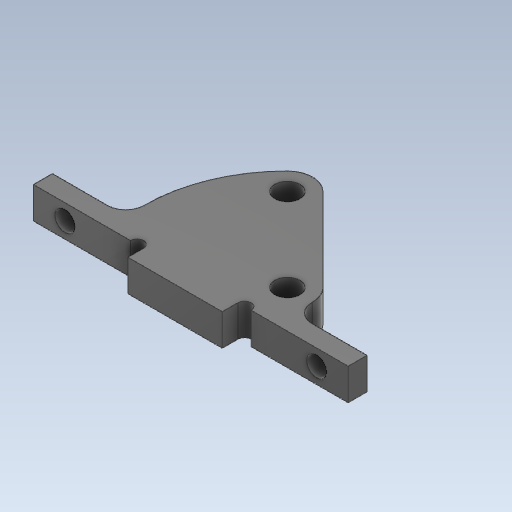
# Autodesk Inventor part: Camera_side_frame
Saved by Autodesk Inventor 2020.4 (Build 244396000, 396)
## iProperties
Part Number: Camera_side_frame
Material: アセタール樹脂、黒
Document SubType Name: Modeling
Designer: Masato Kubotera
Density: 1.425 g/cm^3
Appearance: 滑らか - 黒
Mass: 4.21188 g
Surface Area: 20.6112 cm^2
Volume: 2.95571 cm^3
Description: POM T5
Author: Masato Kubotera
Autodesk Inventor part; units mm, degrees
ref_plane "YZ Plane" through (0, 0, 0) normal (1, 0, 0) x (0, 1, 0)
ref_plane "XZ Plane" through (0, 0, 0) normal (0, 1, 0) x (-1, 0, 0)
ref_plane "XY Plane" through (0, 0, 0) normal (0, 0, 1) x (1, 0, 0)
derived "Head_basis.ipt"
sketch "スケッチ1" plane through (0, 0, 0) normal (0, 1, 0) x (-1, 0, 0)
  line L0 (-44.985, 68.48) -> (-70.7944, 42.6706) construction
  line L1 (4.795, 25.7) -> (-9.205, 25.7) construction
  line L2 (-2.205, 25.7) -> (-44.985, 68.48) construction
  line L3 (-2.205, 25.7) -> (-2.205, 4.9887) construction
  line L4 (-54.1774, 48.681) -> (-57.7129, 52.2165) construction
  line L5 (-57.7129, 52.2165) -> (-80.3403, 29.5891) construction
  line L6 (-80.3403, 29.5891) -> (-76.8048, 26.0536) construction
  line L7 (-76.8048, 26.0536) -> (-54.1774, 48.681) construction
  line L8 (-54.1774, 48.681) -> (-80.3403, 29.5891) construction
  line L9 (-57.7129, 52.2165) -> (-76.8048, 26.0536) construction
  line L10 (-61.9555, 44.4383) -> (-72.5621, 33.8317) construction
  line L11 (-70.7944, 32.064) -> (-60.1878, 42.6706) construction
  circle A0 centre (-59.4807, 46.9132) radius 1.6 construction
  line L12 (-55.9451, 50.4487) -> (-78.5725, 27.8213) construction
  line L13 (17.795, -2.5) -> (-22.205, -2.5) construction
  line L14 (3.8601, -2.5) -> (3.8601, 2.5) construction
  line L15 (5.295, -2.5) -> (5.295, 0)
  line L16 (10.8483, 2.5) -> (7.6861, 2.5) construction
  line L17 (-9.705, -2.5) -> (-9.705, 0)
  line L18 (5.6869, 2.5) -> (7.6861, 2.5) construction
  line L19 (-18.705, 0.5) -> (-16.205, 0.5) construction
  line L20 (-24.705, -2.5) -> (20.295, -2.5) construction
  arc A1 (5.295, -2.5) -> (7.395, -2.5) centre (6.345, -2.5) ccw
  line L21 (9.935, -2.5) -> (11.935, -2.5) construction
  line L22 (7.395, -2.5) -> (22.795, -2.5)
  line L23 (22.795, -2.5) -> (22.795, -5.5)
  line L24 (22.795, -5.5) -> (14.045, -5.5)
  line L25 (17.795, -2.5) -> (17.795, -5.5) construction
  arc A2 (-11.805, -2.5) -> (-9.705, -2.5) centre (-10.755, -2.5) ccw
  line L26 (-11.805, -2.5) -> (-27.205, -2.5)
  line L27 (-27.205, -2.5) -> (-27.205, -5.5)
  line L28 (-22.205, -2.5) -> (-22.205, -5.5) construction
  line L29 (-18.455, -5.5) -> (-27.205, -5.5)
  circle A3 centre (-11.5482, -8.5) radius 2
  arc A4 (14.045, -5.5) -> (11.1379, -8.4177) centre (14.045, -8.4071) ccw
  line L30 (15.045, -5.5) -> (15.045, -6.9) construction
  line L31 (15.045, -6.9) -> (20.545, -6.9) construction
  line L32 (20.545, -5.5) -> (20.545, -6.9) construction
  circle A5 centre (-11.5482, -8.5) radius 4
  line L33 (22.795, -2.5) -> (22.795, 0.5)
  line L34 (-2.205, -12.0113) -> (-2.205, 4.9887) construction
  line L35 (-19.455, -5.5) -> (-19.455, -6.9) construction
  line L36 (-19.455, -6.9) -> (-24.955, -6.9) construction
  line L37 (-24.955, -5.5) -> (-24.955, -6.9) construction
  line L38 (-69.0266, 40.9028) -> (-65.4911, 37.3673) construction
  circle A6 centre (-75.037, 31.3569) radius 1.6
  line L39 (-32.205, -2.5) -> (-22.205, -2.5)
  circle A7 centre (1.665, -21.7132) radius 2
  arc A8 (4.4934, -24.5416) -> (11.1379, -8.4177) centre (-11.5482, -8.5) ccw
  line L40 (-14.3767, -11.3284) -> (-1.1635, -24.5416)
  circle A9 centre (1.665, -21.7132) radius 4
  line L41 (4.4934, -18.8848) -> (-8.7198, -5.6716)
  line L42 (1.665, -21.7132) -> (-11.5482, -8.5) construction
  line L43 (-49.2969, -22.1777) -> (-31.6192, -4.5) construction
  line L44 (-31.6192, -4.5) -> (-28.0837, -8.0355) construction
  line L45 (-28.0837, -8.0355) -> (-45.7614, -25.7132) construction
  line L46 (-45.7614, -25.7132) -> (-49.2969, -22.1777) construction
  line L47 (-49.2969, -22.1777) -> (-28.0837, -8.0355) construction
  line L48 (-31.6192, -4.5) -> (-45.7614, -25.7132) construction
  line L49 (-47.5291, -23.9454) -> (-29.8515, -6.2678) construction
  line L50 (-40.4581, -13.3388) -> (-36.9225, -16.8744) construction
  line L51 (-40.1045, -20.0563) -> (-33.7405, -13.6924) construction
  line L52 (-33.7405, -13.6924) -> (-37.2761, -10.1569) construction
  line L53 (-37.2761, -10.1569) -> (-43.64, -16.5208) construction
  line L54 (-43.64, -16.5208) -> (-40.1045, -20.0563) construction
  line L55 (-40.1045, -20.0563) -> (-37.2761, -10.1569) construction
  line L56 (-33.7405, -13.6924) -> (-43.64, -16.5208) construction
  circle A10 centre (-45.4078, -21.8241) radius 1.6
  line L57 (-42.2258, -15.0359) -> (-38.761, -11.5711)
  line L58 (-37.2761, -10.0861) -> (-33.6698, -13.6924)
  line L59 (-35.1548, -15.1773) -> (-38.6196, -18.6421)
  line L60 (-40.1045, -20.1271) -> (-43.7107, -16.5208)
  line L61 (-43.7107, -16.5208) -> (-33.6698, -13.6924) construction
  line L62 (-37.2761, -10.0861) -> (-40.1045, -20.1271) construction
  arc A11 (-42.2258, -15.0359) -> (-43.7107, -16.5208) centre (-42.9683, -15.7784) ccw
  arc A12 (-37.2761, -10.0861) -> (-38.761, -11.5711) centre (-38.0185, -10.8286) ccw
  circle A13 centre (-31.9728, -8.3891) radius 1.6
  line L63 (-41.8723, -18.2886) -> (-35.5083, -11.9246) construction
  arc A14 (-40.1045, -20.1271) -> (-38.6196, -18.6421) centre (-39.362, -19.3846) ccw
  arc A15 (-35.1548, -15.1773) -> (-33.6698, -13.6924) centre (-34.4123, -14.4349) ccw
  line L64 (-32.205, 19.5) -> (-24.205, 27.5)
  circle A16 centre (-32.205, -2.5) radius 1 construction
  line L65 (-11.5482, -4.5) -> (-31.6192, -4.5)
  line L66 (-57.7129, 52.2165) -> (-54.1774, 48.681)
  line L67 (-76.8048, 26.0536) -> (-80.3403, 29.5891)
  line L68 (-80.3403, 29.5891) -> (-57.7129, 52.2165)
  line L69 (-45.7614, -25.7132) -> (1.665, -25.7132)
  line L70 (-45.7614, -25.7132) -> (-49.2969, -22.1777)
  arc A17 (-15.5479, -8.4464) -> (-18.455, -5.5) centre (-18.455, -8.4074) ccw
  line L71 (-49.2969, 13.1777) -> (-45.7614, 9.6421) construction
  line L72 (-45.7614, 9.6421) -> (-63.439, -8.0355) construction
  line L73 (-49.2969, 13.1777) -> (-63.439, -8.0355) construction
  arc A18 (-59.9035, 2.6418) -> (-61.3884, 1.1569) centre (-60.646, 1.8993) ccw
  line L74 (-52.8324, 2.5004) -> (-56.2972, -0.9645)
  line L75 (-57.7822, -2.4494) -> (-61.3884, 1.1569)
  line L76 (-61.3177, 1.1569) -> (-57.7822, -2.3787) construction
  line L77 (-66.9746, -4.5) -> (-49.2969, 13.1777) construction
  line L78 (-58.1357, 4.3388) -> (-54.6002, 0.8033) construction
  arc A19 (-57.7822, -2.4494) -> (-56.2972, -0.9645) centre (-57.0397, -1.7069) ccw
  line L79 (-59.5499, -0.6109) -> (-53.186, 5.753) construction
  line L80 (-59.9035, 2.6418) -> (-56.4387, 6.1066)
  line L81 (-51.4182, 3.9853) -> (-61.3177, 1.1569) construction
  line L82 (-61.3884, 1.1569) -> (-51.3475, 3.9853) construction
  arc A20 (-52.8324, 2.5004) -> (-51.3475, 3.9853) centre (-52.09, 3.2428) ccw
  line L83 (-57.7822, -2.3787) -> (-51.4182, 3.9853) construction
  line L84 (-54.9537, 7.5208) -> (-61.3177, 1.1569) construction
  arc A21 (-54.9537, 7.5915) -> (-56.4387, 6.1066) centre (-55.6962, 6.8491) ccw
  line L85 (-57.7822, -2.3787) -> (-54.9537, 7.5208) construction
  line L86 (-51.4182, 3.9853) -> (-54.9537, 7.5208) construction
  line L87 (-54.9537, 7.5915) -> (-51.3475, 3.9853)
  circle A22 centre (-49.6504, 9.2886) radius 1.6
  line L88 (-66.9746, -4.5) -> (-45.7614, 9.6421) construction
  line L89 (-65.2068, -6.2678) -> (-47.5291, 11.4099) construction
  line L90 (-54.9537, 7.5915) -> (-57.7822, -2.4494) construction
  line L91 (-63.439, -8.0355) -> (-66.9746, -4.5) construction
  circle A23 centre (-63.0855, -4.1464) radius 1.6
  line L92 (-63.439, -8.0355) -> (-66.9746, -4.5)
  line L93 (-31.6192, -4.5) -> (-45.7614, 9.6421)
  line L94 (-49.2969, 13.1777) -> (-45.7614, 9.6421)
  line L95 (-49.2969, 13.1777) -> (-54.1774, 48.681)
  line L96 (-76.8048, 26.0536) -> (-66.9746, -4.5)
  line L97 (-63.439, -8.0355) -> (-49.2969, -22.1777)
  line L98 (-54.1774, 48.681) -> (-76.8048, 26.0536) construction
  line L99 (-57.2115, 34.0383) -> (-54.7238, 15.9412)
  line L100 (-55.291, 14.2547) -> (-62.4067, 7.139)
  line L101 (-65.7248, 7.9406) -> (-70.7355, 23.5147)
  line L102 (-70.2458, 25.5414) -> (-60.6071, 35.1802)
  arc A24 (-57.2115, 34.0383) -> (-60.6071, 35.1802) centre (-59.1929, 33.7659) ccw
  arc A25 (-70.2458, 25.5414) -> (-70.7355, 23.5147) centre (-68.8316, 24.1272) ccw
  arc A26 (-65.7248, 7.9406) -> (-62.4067, 7.139) centre (-63.8209, 8.5532) ccw
  arc A27 (-55.291, 14.2547) -> (-54.7238, 15.9412) centre (-56.7052, 15.6689) ccw
  line L103 (-15.4772, -17.299) -> (-21.4624, -11.3138)
  line L104 (-24.2908, -11.3138) -> (-30.2761, -17.299)
  line L105 (-28.8619, -20.7132) -> (-16.8914, -20.7132)
  arc A28 (-16.8914, -20.7132) -> (-15.4772, -17.299) centre (-16.8914, -18.7132) ccw
  arc A29 (-21.4624, -11.3138) -> (-24.2908, -11.3138) centre (-22.8766, -12.728) ccw
  arc A30 (-30.2761, -17.299) -> (-28.8619, -20.7132) centre (-28.8619, -18.7132) ccw
  line L106 (-40.1045, -3.0858) -> (-44.3471, 1.1569)
  line L107 (-47.1756, 1.1569) -> (-54.9537, -6.6213)
  line L108 (-54.9537, -9.4497) -> (-50.7111, -13.6924)
  line L109 (-47.8827, -13.6924) -> (-40.1045, -5.9142)
  arc A31 (-40.1045, -5.9142) -> (-40.1045, -3.0858) centre (-41.5187, -4.5) ccw
  arc A32 (-44.3471, 1.1569) -> (-47.1756, 1.1569) centre (-45.7614, -0.2574) ccw
  arc A33 (-54.9537, -6.6213) -> (-54.9537, -9.4497) centre (-53.5395, -8.0355) ccw
  arc A34 (-50.7111, -13.6924) -> (-47.8827, -13.6924) centre (-49.2969, -12.2782) ccw
  circle A35 centre (-11.5482, -8.5) radius 1.6
  circle A36 centre (1.665, -21.7132) radius 1.6
  line L110 (-61.2484, 41.6099) -> (-69.7337, 33.1246) construction
  line L111 (-69.7337, 33.1246) -> (-71.5015, 34.8924) construction
  line L112 (-71.5015, 34.8924) -> (-63.0162, 43.3777) construction
  line L113 (-63.0162, 43.3777) -> (-61.2484, 41.6099) construction
  line L114 (-61.2484, 41.6099) -> (-71.5015, 34.8924) construction
  line L115 (-69.7337, 33.1246) -> (-63.0162, 43.3777) construction
  line L116 (-62.1323, 42.4938) -> (-70.6176, 34.0085) construction
  line L117 (-61.1777, 41.6099) -> (-63.0162, 43.4484)
  line L118 (-63.0162, 43.4484) -> (-71.5722, 34.8924)
  line L119 (-71.5722, 34.8924) -> (-69.7337, 33.0539)
  line L120 (-69.7337, 33.0539) -> (-61.1777, 41.6099)
  line L121 (-61.1777, 41.6099) -> (-71.5722, 34.8924) construction
  line L122 (-63.0162, 43.4484) -> (-69.7337, 33.0539) construction
  arc A37 (-62.6626, 40.125) -> (-61.1777, 41.6099) centre (-61.9202, 40.8674) ccw
  arc A38 (-61.9662, 42.3984) -> (-64.0662, 42.3984) centre (-63.0162, 42.3984) ccw
  arc A39 (-69.7337, 33.0539) -> (-68.2488, 34.5388) centre (-68.9912, 33.7964) ccw
  arc A40 (-70.5222, 35.9424) -> (-70.5222, 33.8424) centre (-70.5222, 34.8924) ccw
  line L123 (-11.955, 0) -> (-15.8241, 0)
  line L124 (-9.705, 0) -> (5.295, 0)
  line L125 (-8.2701, 0) -> (3.8601, 0)
  point P0 (0, 0)
  point P1 (-67.2588, 39.135)
  point P2 (-14.345, -2.5)
  point P3 (-9.705, -2.5)
  point P4 (-14.305, -2.5)
  point P5 (9.895, -2.5)
  point P6 (-38.6903, -15.1066)
  point P7 (-38.6903, -15.1066)
  point P8 (-56.368, 2.5711)
  point P9 (-56.368, 2.5711)
  point P10 (-54.5885, 14.9571)
  point P11 (-66.3749, 38.2511)
  point P12 (-66.3749, 38.2511)
  point P13 (-12.0145, 0)
  point P14 (7.795, -2.5)
  dimension "d5" = 5
  measures "d5" distance of L13.start L22.end
extrude "押し出し1" add sketch "スケッチ1" along normal blind 5 contours A1 L22 L23 L24 A4 A8 A9 L41 A5 L65 L27 L26 A2 L17 L124 L15 | A9 | L40 A5 L41 A9 | L65 A5 A17 L29 L27 | A5
sketch "スケッチ2" plane through (-22.795, 0, -2.5) normal (0, 0, 1) x (1, 0, 0)
  line L0 (0, 0) -> (15.4, 0) projected
  line L1 (5, 0) -> (5, 5) construction
  line L2 (25, 0) -> (25, 5) construction
  line L3 (0, 5) -> (15.4, 5) construction
  line L4 (25, 5) -> (25, 0)
  line L5 (17.5, 5) -> (32.5, 5) projected
  point P0 (5, 2.5)
  point P1 (45, 2.5)
  dimension "d4" = 5
  constraints: 6 end point, 2 midpoint, 2 perpendicular, 2 point on line, 2 symmetric about line, 1 vertical
  measures "d4" distance of L0.start L1.start
hole "穴1" at (-17.795, 2.5, -2.5) at (22.205, 2.5, -2.5) direction (0, 0, -1) diameter 3.2 end through all
equation "\"d4\" = d5"
